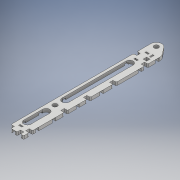
# Autodesk Inventor part: turtlebot_installation_bottom_left
Saved by Autodesk Inventor 2018 (Build 220112000, 112)
## iProperties
Created: 2018-07-15
Part Number: turtlebot_installation_bottom_left
Material: Generic
Document SubType Name: Modeling
Designer: Tsche
Density: 1 g/cm^3
Appearance: Default
Author: Tsche
Autodesk Inventor part; units mm, degrees
ref_plane "YZ Plane" through (0, 0, 0) normal (1, 0, 0) x (0, 1, 0)
ref_plane "XZ Plane" through (0, 0, 0) normal (0, 1, 0) x (-1, 0, 0)
ref_plane "XY Plane" through (0, 0, 0) normal (0, 0, 1) x (1, 0, 0)
sketch "Sketch1" plane through (0, 0, 0) normal (0, 0, 1) x (1, 0, 0)
  circle A0 centre (0, -21) radius 2.1
  circle A1 centre (0, 73) radius 2.1
  line L0 (10, -60.1) -> (10, -55.1)
  line L1 (-5, 73) -> (-5, 60.1)
  line L2 (7, -87.3043) -> (7, -60.1) construction
  line L3 (-5, -56.9) -> (-1.8, -56.9)
  line L4 (10, 68) -> (4, 76)
  arc A2 (4, 76) -> (-5, 73) centre (0, 73) ccw
  line L5 (0.75, 47.5) -> (0.75, -12) construction
  line L6 (4, 47.5) -> (4, -12)
  line L7 (-2.5, -12) -> (-2.5, 47.5)
  arc A3 (4, 47.5) -> (-2.5, 47.5) centre (0.75, 47.5) ccw
  arc A4 (-2.5, -12) -> (4, -12) centre (0.75, -12) ccw
  line L8 (0.75, -30) -> (0.75, -47.5) construction
  line L9 (4, -30) -> (4, -47.5)
  line L10 (-2.5, -47.5) -> (-2.5, -30)
  arc A5 (4, -30) -> (-2.5, -30) centre (0.75, -30) ccw
  arc A6 (-2.5, -47.5) -> (4, -47.5) centre (0.75, -47.5) ccw
  line L11 (-5, 60.1) -> (-2, 60.1)
  line L12 (-2, 60.1) -> (-2, 56.9)
  line L13 (-2, 56.9) -> (-5, 56.9)
  line L14 (7.1, 56.9) -> (3.9, 56.9)
  line L15 (3.9, 56.9) -> (3.9, 60.1)
  line L16 (3.9, 60.1) -> (7.1, 60.1)
  line L17 (2.25, 52.7) -> (-0.75, 52.7)
  line L18 (-0.75, 52.7) -> (-0.75, 54)
  line L19 (2.25, 54) -> (2.25, 52.7)
  line L20 (-0.75, 63) -> (-0.75, 64.3)
  line L21 (-0.75, 64.3) -> (2.25, 64.3)
  line L22 (2.25, 64.3) -> (2.25, 63)
  line L23 (2.25, -54) -> (-0.75, -54)
  line L24 (-0.75, -54) -> (-0.75, -52.7)
  line L25 (-0.75, -52.7) -> (2.25, -52.7)
  line L26 (2.25, -52.7) -> (2.25, -54)
  line L27 (2.25, 54) -> (-0.75, 54)
  line L28 (-0.75, 54) -> (-0.75, 63) construction
  line L29 (-0.75, 63) -> (2.25, 63)
  line L30 (2.25, 63) -> (2.25, 54) construction
  line L31 (2.25, -54) -> (-0.75, -54)
  line L32 (-0.75, -54) -> (-0.75, -60.1) construction
  line L33 (2.25, -60.1) -> (2.25, -54) construction
  circle A7 centre (0, -21) radius 4 construction
  line L34 (10, 55.1) -> (6.9, 55.1)
  line L35 (6.9, 51.9) -> (10, 51.9)
  line L36 (10, 49) -> (4, 49) construction
  line L37 (4, 49) -> (4, 46) construction
  line L38 (4, 46) -> (10, 46) construction
  line L39 (10, 46) -> (10, 49) construction
  line L40 (-5, 0) -> (-73, 0) construction
  line L41 (-5, -60.1) -> (-1.8, -60.1) construction
  line L42 (-1.8, -60.1) -> (-1.8, -56.9)
  line L43 (-5, -56.9) -> (-5, -60.1) construction
  line L44 (3.9, -60.1) -> (3.9, -56.9)
  line L45 (3.9, -56.9) -> (7.1, -56.9)
  line L46 (-1.8, -58.5) -> (3.9, -58.5) construction
  line L47 (3.9, -60.1) -> (-1.8, -60.1)
  line L48 (3.9, -60.1) -> (-1.8, -60.1)
  line L49 (-1.8, -56.9) -> (3.9, -56.9) construction
  line L50 (-5, 56.9) -> (-5, -56.9)
  line L51 (-2, 58.5) -> (3.9, 58.5) construction
  line L52 (-2, 60.1) -> (3.9, 60.1) construction
  line L53 (-2, 56.9) -> (3.9, 56.9) construction
  line L54 (7.1, 60.1) -> (7.1, 56.9)
  line L55 (5.5, 60.1) -> (5.5, 56.9) construction
  line L56 (7.1, -56.9) -> (7.1, -60.1)
  line L57 (7.1, -60.1) -> (10, -60.1)
  line L58 (3.9, -60.1) -> (7.1, -60.1) construction
  line L59 (5.5, -60.1) -> (5.5, -56.9) construction
  line L60 (10, 51.9) -> (10, 55.1) construction
  line L61 (10, 55.1) -> (10, 68)
  line L62 (6, 65) -> (4.7, 65)
  line L63 (4.7, 65) -> (4.7, 62)
  line L64 (4.7, 62) -> (6, 62)
  line L65 (6, 62) -> (6, 65)
  line L66 (4.7, 63.5) -> (6, 63.5) construction
  line L67 (6, 62) -> (10, 62) construction
  line L68 (6, 65) -> (10, 65) construction
  line L69 (4, 46) -> (4, 49) construction
  line L70 (4, 47.5) -> (10, 47.5) construction
  line L71 (6.9, 51.9) -> (6.9, 55.1)
  line L72 (6.9, 53.5) -> (10, 53.5) construction
  line L73 (10, 25.85) -> (6.9, 25.85)
  line L74 (6.9, 22.65) -> (10, 22.65)
  line L75 (10, 22.65) -> (10, 25.85) construction
  line L76 (6.9, 22.65) -> (6.9, 25.85)
  line L77 (6.9, 24.25) -> (10, 24.25) construction
  line L78 (10, 1.6) -> (6.9, 1.6)
  line L79 (6.9, -1.6) -> (10, -1.6)
  line L80 (10, -1.6) -> (10, 0) construction
  line L81 (6.9, -1.6) -> (6.9, 1.6)
  line L82 (6.9, 0) -> (10, 0) construction
  line L83 (10, -19.4) -> (6.9, -19.4)
  line L84 (6.9, -22.6) -> (10, -22.6)
  line L85 (10, -22.6) -> (10, -19.4) construction
  line L86 (6.9, -22.6) -> (6.9, -19.4)
  line L87 (6.9, -21) -> (10, -21) construction
  line L88 (10, -51.9) -> (6.9, -51.9)
  line L89 (6.9, -55.1) -> (10, -55.1)
  line L90 (10, -55.1) -> (10, -51.9) construction
  line L91 (6.9, -55.1) -> (6.9, -51.9)
  line L92 (6.9, -53.5) -> (10, -53.5) construction
  line L93 (10, -46) -> (4, -46) construction
  line L94 (4, -46) -> (4, -49) construction
  line L95 (4, -49) -> (10, -49) construction
  line L96 (10, -49) -> (10, -46) construction
  line L97 (4, -49) -> (4, -46) construction
  line L98 (4, -47.5) -> (10, -47.5) construction
  line L99 (10, -30.5) -> (4, -30.5) construction
  line L100 (4, -30.5) -> (4, -33.5) construction
  line L101 (4, -33.5) -> (10, -33.5) construction
  line L102 (10, -33.5) -> (10, -30.5) construction
  line L103 (4, -33.5) -> (4, -30.5) construction
  line L104 (4, -32) -> (10, -32) construction
  line L105 (4, -11.5) -> (10, -11.5) construction
  line L106 (4, -8.5) -> (4, -11.5) construction
  line L107 (10, -11.5) -> (10, -8.5) construction
  line L108 (10, -8.5) -> (4, -8.5) construction
  line L109 (4, -10) -> (10, -10) construction
  line L110 (4, -11.5) -> (4, -8.5) construction
  line L111 (10, 13.625) -> (4, 13.625) construction
  line L112 (4, 12.125) -> (10, 12.125) construction
  line L113 (10, 10.625) -> (10, 13.625) construction
  line L114 (4, 13.625) -> (4, 10.625) construction
  line L115 (4, 10.625) -> (4, 13.625) construction
  line L116 (4, 10.625) -> (10, 10.625) construction
  line L117 (10, 25.85) -> (10, 51.9)
  line L118 (10, 0) -> (10, 1.6) construction
  line L119 (10, 1.6) -> (10, 22.65)
  line L120 (10, -19.4) -> (10, -1.6)
  line L121 (10, -51.9) -> (10, -22.6)
  line L122 (-89.6, 0) -> (26.6, 0) construction
  line L123 (0, -120.6139) -> (0, 112.553) construction
  line L124 (-2.5, -46) -> (-5, -46) construction
  line L125 (-2.5, -49) -> (-5, -49) construction
  line L126 (-2.5, -33.5) -> (-5, -33.5) construction
  line L127 (-2.5, -30.5) -> (-5, -30.5) construction
  line L128 (-2.5, -11.5) -> (-5, -11.5) construction
  line L129 (-2.5, -8.5) -> (-5, -8.5) construction
  line L130 (-2.5, 49) -> (-5, 49) construction
  line L131 (-2.5, 46) -> (-5, 46) construction
  point P0 (0, 0)
  point P1 (0, 0)
  point P2 (0.75, 17.75)
  point P3 (0.75, -38.75)
  dimension "d0" = 4.2
  dimension "d1" = 4.2
  dimension "d2" = 10
  dimension "d3" = 5
  dimension "d9" = 3.2
  dimension "d11" = 5
  dimension "d12" = 3
  dimension "d13" = 3.2
  dimension "d14" = 8
  dimension "d15" = 3.2
  dimension "d17" = 2.5
  dimension "d19" = 9
  dimension "d20" = 9
  dimension "d25" = 1.5
  dimension "d28" = 1.3
  dimension "d29" = 21
  dimension "d32" = 58.5
  dimension "d34" = 58.5
  dimension "d35" = 3.2
  dimension "d36" = 1.5
  dimension "d38" = 1.5
  dimension "d39" = 11
  dimension "d40" = 11
  dimension "d43" = 4.5
  dimension "d44" = 3
  dimension "d46" = 3
  dimension "d47" = 1.3
  dimension "d48" = 1
  dimension "d49" = 5
  dimension "d50" = 1.3
  dimension "d51" = 3
  dimension "d52" = 4.5
  dimension "d53" = 4.5
  dimension "d54" = 3
  dimension "d55" = 11
  dimension "d57" = 5
  dimension "d58" = 0.1
  dimension "d59" = 3.2
  dimension "d60" = 3.2
  dimension "d61" = 3.2
  dimension "d62" = 3.2
  dimension "d63" = 3.1
  dimension "d64" = 3.1
  dimension "d65" = 3.1
  dimension "d66" = 3.1
  dimension "d67" = 5
  dimension "d68" = 3
  dimension "d69" = 11
  dimension "d70" = 0
  dimension "d72" = 3
  dimension "d73" = 11
  dimension "d74" = 3
  dimension "d75" = 11
  dimension "d77" = 3
  dimension "d81" = 73
  dimension "d82" = 10
  dimension "d92" = 12.125
  dimension "d93" = 24.25
  dimension "d94" = 6
  constraints: 262 end point, 56 collinear, 31 midpoint, 30 parallel, 29 horizontal, 27 point on line, 20 vertical, 15 perpendicular, 10 point on circle, 10 tangent, 8 centre point, 4 coincident, 4 equal length, 14 other
  measures "d0" diameter of A0
  measures "d1" diameter of A1
  measures "d2" distance from line of A0.centre L0
  measures "d3" distance from line of point (0, -21) L1
  measures "d9" distance of L41.start L3.start
  measures "d11" vertical distance of L4.start point (0, 73)
  measures "d12" distance of L12.end L13.end
  measures "d13" distance of L15.end L16.end
  measures "d14" diameter of A7
  measures "d15" distance of L35.start L34.end
  measures "d17" distance between parallel lines of L1 L7
  measures "d19" vertical distance of L5.end A0.centre
  measures "d20" vertical distance of L8.start point (0, -21)
  measures "d25" distance between parallel lines of L30 L5
  measures "d28" distance between parallel lines of L23 L25
  measures "d29" distance from line of L40 point (0, -21)
  measures "d32" distance between parallel lines of L40 L46
  measures "d34" distance between parallel lines of L40 L51
  measures "d35" distance between parallel lines of L11 L13
  measures "d36" distance between parallel lines of L55 L2
  measures "d38" distance between parallel lines of L2 L59
  measures "d39" distance from line of L5.start L51
  measures "d40" distance from line of L46 L8.end
  measures "d43" distance between parallel lines of L23 L46
  measures "d44" distance between parallel lines of L0 L2
  measures "d46" distance of L62.end L63.end
  measures "d47" distance of L62.start L62.end
  measures "d48" distance between parallel lines of L65 L2
  measures "d49" distance between parallel lines of L51 L66
  measures "d50" distance of L20.start L20.end
  measures "d51" distance of L20.end L21.end
  measures "d52" distance between parallel lines of L51 L29
  measures "d53" distance between parallel lines of L51 L27
  measures "d54" distance between parallel lines of L36 L38
  measures "d55" distance between parallel lines of L51 L70
  measures "d57" distance between parallel lines of L51 L72
  measures "d58" distance between parallel lines of L2 L71
  measures "d59" distance of L74.start L73.end
  measures "d60" distance of L79.start L78.end
  measures "d61" distance of L84.start L83.end
  measures "d62" distance of L89.start L88.end
  measures "d63" distance of L89.start L0.end
  measures "d64" distance of L84.start L84.end
  measures "d65" distance of L79.start L79.end
  measures "d66" distance of L74.start L74.end
  measures "d67" distance between parallel lines of L46 L92
  measures "d68" distance between parallel lines of L93 L95
  measures "d69" distance between parallel lines of L46 L98
  measures "d70" distance from line of L87 A0.centre
  measures "d72" distance between parallel lines of L99 L101
  measures "d73" distance from line of point (0, -21) L104
  measures "d74" distance between parallel lines of L108 L105
  measures "d75" distance from line of L109 A0.centre
  measures "d77" distance between parallel lines of L111 L116
  measures "d81" distance from line of A2.centre L40
  measures "d82" distance from line of L117 A1.centre
  measures "d92" distance between parallel lines of L77 L112
  measures "d93" distance between parallel lines of L77 L82
  measures "d94" distance between parallel lines of L6 L119
extrude "Extrusion1" add sketch "Sketch1" along normal blind 3
sketch "Sketch2" plane through (0, 0, 0) normal (0, 0, 1) x (1, 0, 0)
  line L0 (2.25, -60.1) -> (2.25, -54) projected
  line L1 (-0.75, -54) -> (-0.75, -60.1) projected
  line L2 (2.25, -54) -> (-0.75, -54) projected
  line L3 (4, -49) -> (10, -49) projected
  line L4 (10, -46) -> (4, -46) projected
  line L5 (10, -49) -> (10, -46) projected
  line L6 (4, -33.5) -> (10, -33.5) projected
  line L7 (10, -30.5) -> (4, -30.5) projected
  line L8 (4, -11.5) -> (10, -11.5) projected
  line L9 (10, -8.5) -> (4, -8.5) projected
  line L10 (4, 10.625) -> (10, 10.625) projected
  line L11 (10, 13.625) -> (4, 13.625) projected
  line L12 (10, 49) -> (4, 49) projected
  line L13 (4, 46) -> (10, 46) projected
  line L14 (6, 62) -> (10, 62) projected
  line L15 (6, 65) -> (10, 65) projected
  line L16 (6, 62) -> (6, 65) projected
  line L17 (2.25, 63) -> (2.25, 54) projected
  line L18 (-0.75, 54) -> (-0.75, 63) projected
  line L19 (2.25, 54) -> (-0.75, 54) projected
  line L20 (-0.75, 63) -> (2.25, 63) projected
  line L21 (10, 62) -> (10, 65)
  line L22 (10, 49) -> (10, 46)
  line L23 (4, 13.625) -> (4, 10.625)
  line L24 (10, 10.625) -> (10, 13.625)
  line L25 (4, -11.5) -> (4, -8.5)
  line L26 (10, -8.5) -> (10, -11.5)
  line L27 (4, -30.5) -> (4, -33.5)
  line L28 (10, -33.5) -> (10, -30.5)
  line L29 (-0.75, -60.1) -> (2.25, -60.1)
  line L30 (-2.5, -49) -> (-5, -49) projected
  line L31 (-2.5, -46) -> (-5, -46) projected
  line L32 (-2.5, -33.5) -> (-5, -33.5) projected
  line L33 (-2.5, -30.5) -> (-5, -30.5) projected
  line L34 (-2.5, -11.5) -> (-5, -11.5) projected
  line L35 (-2.5, -8.5) -> (-5, -8.5) projected
  line L36 (-2.5, 46) -> (-5, 46) projected
  line L37 (-2.5, 49) -> (-5, 49) projected
  line L38 (-5, -49) -> (-5, -46)
  line L39 (-2.5, -33.5) -> (-2.5, -30.5)
  line L40 (-5, -33.5) -> (-5, -30.5)
  line L41 (-2.5, -11.5) -> (-2.5, -8.5)
  line L42 (-5, -11.5) -> (-5, -8.5)
  line L43 (-5, 46) -> (-5, 49)
  line L44 (4, -49) -> (-2.5, -49)
  line L45 (4, -46) -> (-2.5, -46)
  line L46 (4, 49) -> (-2.5, 49)
  line L47 (4, 46) -> (-2.5, 46)
  line L48 (-2.5, 47.5) -> (-2.5, -12) projected
  point P0 (0, 0)
  constraints: 38 end point, 9 parallel, 4 perpendicular, 2 collinear, 1 vertical
extrude "Extrusion2" cut sketch "Sketch2" along normal blind 1.3
fillet "Fillet1" radius 1 17 edges at (10, -60.1, 1.5) (3.9, -60.1, 1.5) (7.1, -60.1, 1.5) (10, -55.1, 1.5) (10, -51.9, 1.5) (10, -22.6, 1.5) (10, -19.4, 1.5) (10, -1.6, 1.5) (10, 1.6, 1.5) (10, 22.65, 1.5) (10, 25.85, 1.5) (10, 51.9, 1.5) (10, 55.1, 1.5) (-5, 60.1, 1.5) (-5, 56.9, 1.5) (-1.8, -60.1, 1.5) (-5, -56.9, 1.5)
fillet "Fillet2" radius 5 1 edges at (10, 68, 1.5)
fillet "Fillet3" radius 1.5 16 edges at (0.75, -60.1, 1.3) (0.75, -54, 1.3) (10, -47.5, 1.3) (4, -46.75, 1.3) (10, -32, 1.3) (4, -32, 1.3) (4, -10, 1.3) (10, -10, 1.3) (4, 12.125, 1.3) (10, 12.125, 1.3) (4, 46.75, 1.3) (10, 47.5, 1.3) (6, 63.5, 1.3) (10, 63.5, 1.3) (0.75, 63, 1.3) (0.75, 54, 1.3)
body "Solid1"
